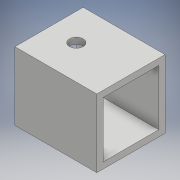
# Autodesk Inventor part: bracket1(body)
Saved by Autodesk Inventor 2018.2 (Build 222227000, 227)
## iProperties
Created: 2018-03-21
Part Number: bracket1(body)
Material: 一般
Document SubType Name: Modeling
Designer: ku_sk
Density: 1 g/cm^3
Appearance: 既定
Author: ku_sk
Autodesk Inventor part; units mm, degrees
ref_plane "YZ Plane" through (0, 0, 0) normal (1, 0, 0) x (0, 1, 0)
ref_plane "XZ Plane" through (0, 0, 0) normal (0, 1, 0) x (-1, 0, 0)
ref_plane "XY Plane" through (0, 0, 0) normal (0, 0, 1) x (1, 0, 0)
sketch "スケッチ1" plane through (0, 0, 0) normal (1, 0, 0) x (0, 1, 0)
  line L0 (-12.5, 12.5) -> (12.5, 12.5)
  line L1 (12.5, 12.5) -> (12.5, -12.5)
  line L2 (12.5, -12.5) -> (-12.5, -12.5)
  line L3 (-12.5, -12.5) -> (-12.5, 12.5)
  line L4 (-12.5, 12.5) -> (12.5, -12.5) construction
  line L5 (12.5, 12.5) -> (-12.5, -12.5) construction
  line L6 (-10.2, 10.2) -> (10.2, 10.2)
  line L7 (10.2, 10.2) -> (10.2, -10.2)
  line L8 (10.2, -10.2) -> (-10.2, -10.2)
  line L9 (-10.2, -10.2) -> (-10.2, 10.2)
  line L10 (-10.2, 10.2) -> (10.2, -10.2) construction
  line L11 (10.2, 10.2) -> (-10.2, -10.2) construction
  point P0 (0, 0)
  dimension "d0" = 25
  dimension "d1" = 25
  dimension "d2" = 2.3
  constraints: 24 end point, 4 midpoint, 4 parallel, 2 horizontal, 2 perpendicular, 1 point on line
  measures "d0" distance of L0.start L0.end
  measures "d1" distance of L0.end L1.end
  measures "d2" distance between parallel lines of L6 L0
extrude "押し出し1" add sketch "スケッチ1" along normal blind 30
sketch "スケッチ2" plane through (0, -12.5, 12.5) normal (0, 0, 1) x (1, 0, 0)
  circle A0 centre (10, 12.5) radius 2.5
  line L0 (0, 0) -> (0, 25) projected
  line L1 (0, 0) -> (30, 0) projected
  point P0 (0, 12.5)
  dimension "d5" = 5
  dimension "d6" = 10
  dimension "d7" = 12.5
  constraints: 1 centre point
  measures "d5" diameter of A0
  measures "d6" distance from line of L0 A0.centre
  measures "d7" distance from line of L1 A0.centre
extrude "押し出し2" cut sketch "スケッチ2" against normal through all
